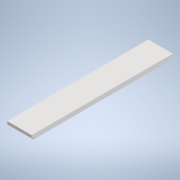
# Autodesk Inventor part: Arcade_top
Saved by Autodesk Inventor 2022 (Build 260153000, 153)
## iProperties
Created: 2023-12-22
Part Number: Arcade_top
Material: Generic
Document SubType Name: Modeling
Designer: Petr Černý
Density: 1 g/cm^3
Appearance: Default
Author: Petr Černý
Autodesk Inventor part; units mm, degrees
ref_plane "YZ Plane" through (0, 0, 0) normal (1, 0, 0) x (0, 1, 0)
ref_plane "XZ Plane" through (0, 0, 0) normal (0, 1, 0) x (-1, 0, 0)
ref_plane "XY Plane" through (0, 0, 0) normal (0, 0, 1) x (1, 0, 0)
sketch "Sketch1" plane through (0, 0, 0) normal (0, 1, 0) x (-1, 0, 0)
  line L0 (28.3692, 74.6141) -> (-56.6308, 74.6141)
  line L1 (-56.6308, 74.6141) -> (-56.6308, -415.3859)
  line L2 (-56.6308, -415.3859) -> (28.3692, -415.3859)
  line L3 (28.3692, -415.3859) -> (28.3692, 74.6141)
  point P0 (0, 0)
  dimension "d0" = 85
  dimension "d1" = 490
  constraints: 8 end point, 2 parallel, 1 horizontal, 1 perpendicular
  measures "d0" distance of L2.end L1.end
  measures "d1" distance of L1.end L0.end
extrude "Extrusion1" add sketch "Sketch1" along normal blind 15
sketch "Sketch2" plane through (-28.3692, 0, 74.6141) normal (0, 0, 1) x (1, 0, 0)
  line L0 (85, 0) -> (0, 0) projected
  line L1 (0, 0) -> (85, 0)
  line L2 (85, 0) -> (85, 5)
  line L3 (85, 5) -> (0, 5)
  line L4 (0, 5) -> (0, 0)
  point P0 (28.3692, 0)
  dimension "d4" = 85
  dimension "d5" = 5
  constraints: 8 end point, 2 parallel, 1 horizontal, 1 perpendicular
  measures "d4" distance of L3.end L2.end
  measures "d5" distance of L2.end L1.end
extrude "Extrusion2" cut sketch "Sketch2" against normal blind 7
sketch "Sketch3" plane through (56.6308, 0, -415.3859) normal (0, 0, -1) x (-1, 0, 0)
  line L0 (85, 0) -> (85, 15) projected
  line L1 (85, 5) -> (0, 5) projected
  line L2 (85, 0) -> (0, 0)
  line L3 (0, 0) -> (0, 5)
  line L4 (0, 5) -> (85, 5)
  line L5 (85, 5) -> (85, 0)
  point P0 (56.6308, 0)
  dimension "d8" = 85
  dimension "d9" = 5
  constraints: 8 end point, 2 parallel, 1 horizontal, 1 perpendicular
  measures "d8" distance of L1.end L4.end
  measures "d9" distance of L2.end L1.end
extrude "Extrusion3" cut sketch "Sketch3" against normal blind 7
sketch "Sketch4" plane through (0, 0, 0) normal (0, -1, 0) x (1, 0, 0)
  line L0 (-28.3692, -408.3859) -> (56.6308, -408.3859) projected
  line L1 (56.6308, 67.6141) -> (56.6308, -408.3859) projected
  line L2 (56.6308, 67.6141) -> (-28.3692, 67.6141) projected
  line L3 (-28.3692, -408.3859) -> (-28.3692, 67.6141) projected
  line L4 (-28.3692, 67.6141) -> (56.6308, 67.6141) projected
  line L5 (-28.3692, -408.3859) -> (-28.3692, 67.6141) projected
  line L6 (56.6308, 67.6141) -> (-28.3692, 67.6141)
  line L7 (-28.3692, 67.6141) -> (-28.3692, -408.3859)
  line L8 (-28.3692, -408.3859) -> (56.6308, -408.3859)
  line L9 (56.6308, -408.3859) -> (56.6308, 67.6141)
  point P0 (0, 0)
  constraints: 8 end point, 2 parallel, 1 horizontal, 1 perpendicular
extrude "Extrusion4" add sketch "Sketch4" along normal blind 1
body "Solid1"
